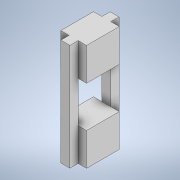
# Autodesk Inventor part: spacer_4
Saved by Autodesk Inventor 2021.2 (Build 252289000, 289)
## iProperties
Created: 2021-03-24
Part Number: spacer_4
Material: Generic
Document SubType Name: Modeling
Designer: yxion
Density: 1 g/cm^3
Appearance: Default
Author: yxion
Autodesk Inventor part; units mm, degrees
ref_plane "YZ Plane" through (0, 0, 0) normal (1, 0, 0) x (0, 1, 0)
ref_plane "XZ Plane" through (0, 0, 0) normal (0, 1, 0) x (-1, 0, 0)
ref_plane "XY Plane" through (0, 0, 0) normal (0, 0, 1) x (1, 0, 0)
sketch "Sketch1" plane through (0, 0, 0) normal (0, 0, 1) x (1, 0, 0)
  line L0 (-18.4125, 60.1579) -> (1.5875, 60.1579)
  line L1 (1.5875, 60.1579) -> (1.5875, 34.7579)
  line L2 (1.5875, 34.7579) -> (-18.4125, 34.7579)
  line L3 (-18.4125, 34.7579) -> (-18.4125, 60.1579)
  line L4 (-18.4125, 3.0079) -> (1.5875, 3.0079)
  line L5 (1.5875, 3.0079) -> (1.5875, -22.3921)
  line L6 (1.5875, -22.3921) -> (-18.4125, -22.3921)
  line L7 (-18.4125, -22.3921) -> (-18.4125, 3.0079)
  point P0 (0, 0)
  dimension "d0" = 25.4
  dimension "d1" = 25.4
  dimension "d2" = 20
  dimension "d5" = 31.75
  constraints: 16 end point, 4 parallel, 2 horizontal, 2 perpendicular, 2 point on line
  measures "d0" distance of L0.end L1.end
  measures "d1" distance of L4.end L5.end
  measures "d2" distance of L0.start L0.end
  measures "d5" distance between parallel lines of L4 L2
extrude "Extrusion1" add sketch "Sketch1" along normal blind 25.4
sketch "Sketch2" plane through (0, 0, 25.4) normal (0, 0, 1) x (1, 0, 0)
  line L0 (1.5875, 60.1579) -> (-18.4125, 60.1579) projected
  line L1 (-18.4125, -22.3921) -> (1.5875, -22.3921) projected
  line L2 (1.5875, 60.1579) -> (-11.9125, 60.1579)
  line L3 (-11.9125, 60.1579) -> (-11.9125, -22.3921)
  line L4 (-11.9125, -22.3921) -> (-4.9125, -22.3921)
  line L5 (-4.9125, -22.3921) -> (-4.9125, 60.1579)
  line L6 (-18.4125, 34.7579) -> (1.5875, 34.7579) projected
  line L7 (1.5875, 34.7579) -> (1.5875, 60.1579) projected
  line L8 (1.5875, 60.1579) -> (-18.4125, 60.1579) projected
  line L9 (-18.4125, 60.1579) -> (-18.4125, 34.7579) projected
  line L10 (-18.4125, -22.3921) -> (1.5875, -22.3921) projected
  line L11 (1.5875, -22.3921) -> (1.5875, 3.0079) projected
  line L12 (1.5875, 3.0079) -> (-18.4125, 3.0079) projected
  line L13 (-18.4125, 3.0079) -> (-18.4125, -22.3921) projected
  point P0 (0, 0)
  point P1 (-11.9125, 34.7579)
  point P2 (-11.9125, 3.0079)
  point P3 (-9.9654, 60.1579)
  dimension "d14" = 20
  dimension "d15" = 7
  dimension "d16" = 6.5
  constraints: 8 end point, 2 parallel, 2 point on line, 1 horizontal, 1 perpendicular
  measures "d14" distance between parallel lines of L7 L9
  measures "d15" distance between parallel lines of L5 L3
  measures "d16" distance between parallel lines of L7 L5
extrude "Extrusion2" add sketch "Sketch2" along normal blind 6.35 contours L5 L6 L3 L0 | L5 L12 L3 L6 | L5 L1 L3 L12
sketch "Sketch3" plane through (0, 0, 0) normal (0, 0, -1) x (-1, 0, 0)
  line L0 (4.9125, 3.0079) -> (11.9125, 3.0079) projected
  line L1 (11.9125, 34.7579) -> (11.9125, 3.0079) projected
  line L2 (11.9125, 34.7579) -> (4.9125, 34.7579) projected
  line L3 (4.9125, 3.0079) -> (4.9125, 34.7579) projected
  line L4 (11.9125, 34.7579) -> (11.9125, 60.1579) projected
  line L5 (4.9125, 60.1579) -> (4.9125, 34.7579) projected
  line L6 (11.9125, -22.3921) -> (11.9125, 3.0079) projected
  line L7 (4.9125, 3.0079) -> (4.9125, -22.3921) projected
  line L8 (11.9125, 60.1579) -> (4.9125, 60.1579)
  line L9 (-1.5875, 60.1579) -> (18.4125, 60.1579) projected
  line L10 (11.9125, -22.3921) -> (4.9125, -22.3921)
  line L11 (18.4125, -22.3921) -> (-1.5875, -22.3921) projected
  point P0 (0, 0)
  constraints: 4 end point, 2 collinear
extrude "Extrusion3" add sketch "Sketch3" along normal blind 6.35
equation "\"d16\" = -0.5 * d15 + 0.5 * d14"
body "Solid1"
